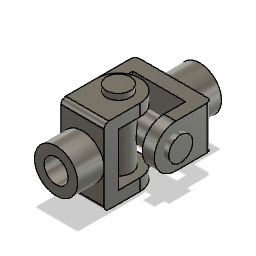
universal joint (Autodesk Fusion 360 design; units mm, degrees)
Autodesk Fusion 360 part; units mm, degrees
sketch "Sketch1" plane through (0, 0, 0) normal (0, 1, 0) x (1, 0, 0)
  circle A0 centre (0, 0) radius 0.3
  dimension "d1" = 0.6
  constraint coincident A0.centre origin
  measures "d1" diameter of A0
extrude "Extrude1" add sketch "Sketch1" along normal blind 3.6 makes body 1 in component "Component"
sketch "Sketch2" plane through (0, 3.6, 0) normal (0, 1, 0) x (-1, 0, 0)
  circle A0 centre (0, 0) radius 0.3
  circle A1 centre (0, 0) radius 0.5
  dimension "d4" = 1
  constraint coincident A0.centre A1.centre
  measures "d4" diameter of A1
extrude "Extrude2" add sketch "Sketch2" against normal blind 0.25 bodies 1 in component "Component"
ref_plane "WorkPlane1" through (0, 1.8, 0) normal (0, -1, 0) x (-1, 0, 0)
mirror "Mirror1" about plane through (0, 1.8, 0) normal (0, -1, 0) of "Extrude2" in component "Component"
sketch "Sketch3" plane through (0, 0, 0) normal (0, 0, 1) x (1, 0, 0)
sketch "Sketch4" plane through (0, 0, 0) normal (0, 0, 1) x (1, 0, 0)
  circle A0 centre (0, 0) radius 0.9
  circle A1 centre (0, 0) radius 0.5
  dimension "d9" = 1.8
  dimension "d10" = 1
  constraint coincident A0.centre A1.centre
  measures "d9" diameter of A0
  measures "d10" diameter of A1
extrude "Extrude1'" add sketch "Sketch4" along normal blind 1.1 separate body makes body 2 in component "Component'"
sketch "Sketch5" plane through (0, 0, 0) normal (0, 0, -1) x (-1, 0, 0)
  circle A0 centre (0, 0) radius 0.5
  circle A1 centre (0, 0) radius 0.9
  line L0 (0.9, -1.6) -> (-0.9, -1.6)
  line L1 (-0.9, -1.6) -> (-0.9, 1.6)
  line L2 (-0.9, 1.6) -> (0.9, 1.6)
  line L3 (0.9, 1.6) -> (0.9, -1.6)
  line L4 (0.9, -1.6) -> (-0.9, 1.6) construction
  line L5 (-0.9, -1.6) -> (0.9, 1.6) construction
  dimension "d13" = 3.2
  dimension "d14" = 1.8
  constraint horizontal L0
  constraint perpendicular L0 L1
  constraint parallel L0 L2
  constraint parallel L1 L3
  constraint coincident L4 A0.centre
  constraint coincident L5 A0.centre
  constraint coincident A0.centre A1.centre
  measures "d13" distance of L0.end L1.end
  measures "d14" distance of L0.start L0.end
extrude "Extrude2'" add sketch "Sketch5" along normal blind 0.6 contours A0 | A1 | A1 L0 L1 L3 | A1 L1 L2 L3 bodies 2 in component "Component'"
sketch "Sketch6" plane through (0, 0, 0) normal (0, 0, -1) x (1, 0, 0)
sketch "Sketch8" plane through (0, 1.6, 0) normal (0, 1, 0) x (-1, 0, 0)
  line L0 (0.9, 0) -> (-0.9, 0)
  line L1 (-0.9, 0) -> (-0.9, -0.6)
  line L2 (-0.9, -0.6) -> (0.9, -0.6)
  line L3 (0.9, -0.6) -> (0.9, 0)
  line L4 (0.9, -0.6) -> (0.9, 0)
  line L5 (0.9, 0) -> (-0.9, 0)
  line L6 (-0.9, 0) -> (-0.9, -0.6)
  line L7 (0.9, 1.1) -> (-0.9, 1.1)
  line L8 (0.9, -0.6) -> (0.9, -1.5)
  line L9 (-0.9, -0.6) -> (-0.9, -1.5)
  circle A0 centre (0, -1.5) radius 0.3
  arc A1 (-0.9, -1.5) -> (0.9, -1.5) centre (0, -1.5) ccw
  line L10 (0.9, -0.6) -> (-0.9, -0.6)
  dimension "d22" = 2.6
  dimension "d23" = 0.6
  constraint coincident L2.end L3.start
  constraint coincident L0.start L3.end
  constraint coincident L0.end L1.start
  constraint coincident L1.end L2.start
  constraint perpendicular L2 L8
  constraint perpendicular L2 L9
  constraint tangent L8 A1
  constraint concentric A0 A1
  measures "d22" distance of L7 L8.end
  measures "d23" diameter of A0
extrude "Extrude3" add sketch "Sketch8" against normal blind 0.5 contours L2 L8 L9 A1 L10 bodies 2 in component "Component'"
ref_plane "WorkPlane2" through (0, 0, -1.2) normal (0, 1, 0) x (1, 0, 0)
mirror "Mirror1'" about plane through (0, 0, -1.2) normal (0, 1, 0) of "Extrude3" in component "Component'"
fillet "Fillet1" radius 0.2 2 edges at (0, 1.6, 0) (0, -1.6, 0) on bodies 2 in component "Component'"
sketch "Sketch9" plane through (0, 0, 0) normal (0, 1, 0) x (1, 0, 0)
  circle A0 centre (0, 0) radius 0.55
  circle A1 centre (0, 0) radius 0.3
  dimension "d30" = 1.1
  dimension "d31" = 0.6
  constraint coincident A0.centre A1.centre
  measures "d30" diameter of A0
  measures "d31" diameter of A1
extrude "Extrude1''" add sketch "Sketch9" along normal blind 2.2 separate body makes body 3 in component "Component''"
ref_plane "WorkPlane3" through (0, 0, 1.1) normal (0, 0, 1) x (1, 0, 0)
ref_plane "WorkPlane4" through (0, 0, -1.1) normal (0, 0, 1) x (1, 0, 0)
sketch "Sketch10" plane through (0, 0, 1.1) normal (0, 0, 1) x (1, 0, 0)
  circle A0 centre (0.8, 1.1) radius 0.55
  circle A1 centre (0.8, 1.1) radius 0.3
  dimension "d36" = 1.1
  dimension "d37" = 0.6
  dimension "d38" = 1.1
  dimension "d39" = 0.8
  constraint concentric A0 A1
  measures "d36" diameter of A0
  measures "d37" diameter of A1
  measures "d38" vertical distance of origin A0.centre
  measures "d39" horizontal distance of origin A0.centre
extrude "Extrude2''" add sketch "Sketch10" against normal blind 2.2 bodies 3 in component "Component''"
copy_body "CopyPasteBodies1" bodies 2 body 2 seen with x (1, 0, 0) y (0, 1, 0) z (0, 0, 1) at (0.1447, -0.3925, 0.47) makes body 4
move_body "Move1" bodies 4 to x (0, 1, 0) y (1, 0, 0) z (0, 0, -1) at (1.1881, -1.1881, -12.1487)
copy_body "Body->Comp1" bodies 4 removing the originals makes body 5 in component "Component'''"
component "Component" placed x (1, 0, 0) y (0, 1, 0) z (0, 0, 1) at (0.1447, -2.1425, -1.03)
component "Component'" placed x (1, 0, 0) y (0, 1, 0) z (0, 0, 1) at (0.1447, -0.3925, 0.47)
component "Component''" placed x (0, 0, -1) y (0, 1, 0) z (1, 0, 0) at (0.1447, -1.4925, -1.03)
component "Component'''" placed x (1, 0, 0) y (0, 1, 0) z (0, 0, 1) at (-0.6509, 0.6509, 9.2887)
component "Component" placed x (0, -1, 0) y (1, 0, 0) z (0, 0, 1) at (-1.6553, -0.3925, -1.83)
